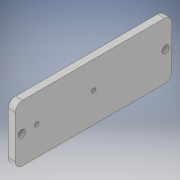
# Autodesk Inventor part: Base Plate.
Saved by Autodesk Inventor 2017.3 (Build 213256000, 256)
## iProperties
Created: 2017-04-14
Part Number: Base Plate.
Material: Generic
Document SubType Name: Modeling
Designer: 167898
Density: 1 g/cm^3
Appearance: Default
Author: 167898
Autodesk Inventor part; units mm, degrees
ref_plane "YZ Plane" through (0, 0, 0) normal (1, 0, 0) x (0, 1, 0)
ref_plane "XZ Plane" through (0, 0, 0) normal (0, 1, 0) x (-1, 0, 0)
ref_plane "XY Plane" through (0, 0, 0) normal (0, 0, 1) x (1, 0, 0)
sketch "Sketch1" plane through (0, 0, 0) normal (1, 0, 0) x (0, 1, 0)
  line L0 (152.1482, 345.366) -> (50.5482, 345.366)
  line L1 (50.5482, 345.366) -> (50.5482, 65.966)
  line L2 (50.5482, 65.966) -> (152.1482, 65.966)
  line L3 (152.1482, 65.966) -> (152.1482, 345.366)
  point P0 (0, 0)
  dimension "d0" = 279.4
  dimension "d1" = 101.6
  constraints: 8 end point, 2 parallel, 1 horizontal, 1 perpendicular
  measures "d0" distance of L2.end L0.start
  measures "d1" distance of L1.end L2.end
extrude "Extrusion1" add sketch "Sketch1" along normal blind 12.7
fillet "Fillet1" radius 12.7 4 edges at (6.35, 152.1482, 345.366) (6.35, 152.1482, 65.966) (6.35, 50.5482, 345.366) (6.35, 50.5482, 65.966)
sketch "Sketch2" plane through (12.7, 0, 0) normal (1, 0, 0) x (0, 0, -1)
  line L0 (-345.366, 139.4482) -> (-345.366, 63.2482) projected
  line L1 (-345.366, 101.3482) -> (-65.966, 101.3482)
  line L2 (-65.966, 63.2482) -> (-65.966, 139.4482) projected
  line L3 (-345.366, 152.1482) -> (-334.254, 152.0486)
  arc A0 (-332.666, 152.1482) -> (-345.366, 139.4482) centre (-332.666, 139.4482) ccw projected
  line L4 (-334.254, 152.0486) -> (-334.254, 101.3482)
  circle A1 centre (-334.254, 101.3482) radius 6.35
  point P0 (0, 0)
  dimension "d5" = 11.1125
  dimension "d6" = 12.7
  constraints: 6 end point, 2 midpoint, 1 centre point, 1 coincident, 1 perpendicular, 1 point on circle, 1 point on line
  measures "d5" distance of L3.start L3.end
  measures "d6" diameter of A1
extrude "Extrusion2" cut sketch "Sketch2" against normal blind 42.8625 contours A1 L4 L1 | L1 A1 | A1 L1 L4
sketch "Sketch3" plane through (12.7, 0, 0) normal (1, 0, 0) x (0, 0, -1)
  line L0 (-345.366, 152.1482) -> (-307.266, 152.1482)
  line L1 (-78.666, 152.1482) -> (-332.666, 152.1482) projected
  line L2 (-307.266, 152.1482) -> (-307.266, 102.2169)
  circle A0 centre (-307.266, 102.2169) radius 3.81
  point P0 (0, 0)
  dimension "d9" = 38.1
  dimension "d10" = 7.62
  constraints: 4 end point, 1 centre point, 1 coincident, 1 perpendicular, 1 point on line
  measures "d9" distance of L0.start L0.end
  measures "d10" diameter of A0
extrude "Extrusion3" cut sketch "Sketch3" against normal blind 88.9
sketch "Sketch4" plane through (12.7, 0, 0) normal (1, 0, 0) x (0, 0, -1)
  line L0 (-65.966, 63.2482) -> (-65.966, 139.4482) projected
  line L1 (-65.966, 103.1393) -> (-299.4746, 103.1393)
  point P0 (0, 0)
  constraints: 2 end point, 1 perpendicular, 1 point on line
sketch "Sketch5" plane through (12.7, 0, 0) normal (1, 0, 0) x (0, 0, -1)
  line L0 (-345.366, 152.1482) -> (-205.666, 152.1482)
  line L1 (-78.666, 152.1482) -> (-332.666, 152.1482) projected
  line L2 (-205.666, 103.8134) -> (-205.666, 152.1482)
  circle A0 centre (-205.666, 103.8134) radius 3.81
  point P0 (0, 0)
  dimension "d13" = 7.62
  constraints: 4 end point, 1 centre point, 1 coincident, 1 midpoint, 1 perpendicular
  measures "d13" diameter of A0
extrude "Extrusion4" cut sketch "Sketch5" against normal blind 214.3125
sketch "Sketch6" plane through (12.7, 0, 0) normal (1, 0, 0) x (0, 0, -1)
  line L0 (-65.966, 152.1482) -> (-77.0785, 152.1482)
  line L1 (-78.666, 152.1482) -> (-332.666, 152.1482) projected
  line L2 (-77.0785, 152.1482) -> (-77.0785, 103.1012)
  circle A0 centre (-77.0785, 103.1012) radius 6.35
  point P0 (0, 0)
  dimension "d16" = 11.1125
  dimension "d17" = 12.7
  constraints: 4 end point, 1 centre point, 1 coincident, 1 collinear, 1 perpendicular
  measures "d16" distance of L0.start L0.end
  measures "d17" diameter of A0
extrude "Extrusion5" cut sketch "Sketch6" against normal blind 211.1375
sketch "Sketch7" plane through (12.7, 0, 0) normal (1, 0, 0) x (0, 0, -1)
  point P0 (0, 0)
body "Solid1"
